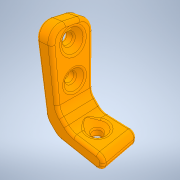
# Autodesk Inventor part: Уголок
Saved by Autodesk Inventor 2021.1 (Build 251245010, 245A)
## iProperties
Created: 2026-06-28
Part Number: Уголок
Material: Типовые
Document SubType Name: Modeling
Designer: Андрей Тарасов
Density: 1 g/cm^3
Appearance: По умолчанию
Author: Андрей Тарасов
Autodesk Inventor part; units mm, degrees
ref_plane "YZ Plane" through (0, 0, 0) normal (1, 0, 0) x (0, 1, 0)
ref_plane "XZ Plane" through (0, 0, 0) normal (0, 1, 0) x (-1, 0, 0)
ref_plane "XY Plane" through (0, 0, 0) normal (0, 0, 1) x (1, 0, 0)
sketch "Эскиз1" plane through (0, 0, 0) normal (0, 0, 1) x (1, 0, 0)
  line L0 (0, 30) -> (0, 0)
  line L1 (0, 0) -> (20, 0)
  line L2 (20, 0) -> (20, 5)
  line L3 (20, 5) -> (5, 5)
  line L4 (5, 5) -> (5, 30)
  line L5 (5, 30) -> (0, 30)
  line L6 (0, 25) -> (5, 25) construction
  line L7 (0, 15) -> (5, 15) construction
  point P0 (0, 0)
  dimension "d0" = 30
  dimension "d1" = 15
  dimension "d2" = 10
  dimension "d3" = 20
  dimension "d4" = 5
  dimension "d5" = 5
  constraints: 16 end point, 5 perpendicular, 3 point on line, 2 horizontal, 1 coincident, 1 midpoint, 1 parallel
  measures "d0" distance between parallel lines of L1 L5
  measures "d1" distance between parallel lines of L1 L7
  measures "d2" distance between parallel lines of L6 L7
  measures "d3" distance between parallel lines of L2 L0
  measures "d4" distance between parallel lines of L3 L1
  measures "d5" distance between parallel lines of L4 L0
extrude "Выдавливание1" add sketch "Эскиз1" along normal blind 12
sketch "Эскиз2" plane through (0, 0, 0) normal (-1, 0, 0) x (0, 0, 1)
  line L0 (0, 30) -> (12, 30) projected
  line L1 (6, 30) -> (6, 0) construction
  line L2 (0, 0) -> (12, 0) projected
  circle A0 centre (6, 15.3) radius 1.6
  circle A1 centre (6, 25.3) radius 1.6
  dimension "d8" = 3.2
  dimension "d9" = 10
  dimension "d10" = 15.3
  constraints: 2 centre point, 2 end point, 2 midpoint, 2 point on line, 1 equal radius
  measures "d8" diameter of A0
  measures "d9" distance of A0.centre A1.centre
  measures "d10" distance from line of L2 A0.centre
extrude "Выдавливание2" cut sketch "Эскиз2" against normal up to surface (5 mm away)
sketch "Эскиз3" plane through (5, 5, 0) normal (0, 1, 0) x (1, 0, 0)
  circle A0 centre (7.5, -6) radius 1.6
  line L0 (0, 0) -> (0, -12) projected
  line L1 (0, -6) -> (15, -6) construction
  line L2 (15, 0) -> (15, -12) projected
  point P0 (-5, 0)
  dimension "d22" = 3.2
  constraints: 3 midpoint, 2 end point, 1 centre point
  measures "d22" diameter of A0
extrude "Выдавливание3" cut sketch "Эскиз3" against normal up to surface (5 mm away)
chamfer "Фаска1" distance 1.8 angle 45 3 edges at (5, 25.3, 4.4) (5, 15.3, 4.4) (10.9, 5, 6)
chamfer "Фаска2" distance 4 angle 45 2 edges at (5, 5, 6) (0, 0, 6)
fillet "Сопряжение1" radius 4 6 edges at (2.5, 30, 12) (2.5, 30, 0) (0, 4, 6) (4, 0, 6) (5, 9, 6) (9, 5, 6)
fillet "Сопряжение1" radius 2 2 edges at (20, 5, 6) (20, 0, 6)
fillet "Сопряжение2" radius 1 37 edges at (3.2, 25.3, 4.4) (0, 25.3, 4.4) (0, 15.8284, 12) (0.3045, 4.1261, 12) (2, 2, 12) (4.1261, 0.3045, 12) (11.8284, 0, 12) (0, 30, 6) (0, 28.8284, 1.1716) (0, 15.8284, 0) (0.3045, 4.1261, 0) (2, 2, 0) (4.1261, 0.3045, 0) (11.8284, 0, 0) (0, 28.8284, 10.8284) (0, 15.3, 4.4) (3.2, 15.3, 4.4) (5, 25.3, 2.6) (5, 15.3, 2.6) (5, 28.8284, 1.1716) (5, 30, 6) (5, 28.8284, 10.8284) (5, 18.3284, 12) (2.5, 26, 12) (7, 7, 12) (19.4142, 4.4142, 12) (14.3284, 5, 12) (2.5, 26, 0) (7, 7, 0) (19.4142, 4.4142, 0) (14.3284, 5, 0) (5, 18.3284, 0) (10.9, 0, 6) (10.9, 3.2, 6) (8.4117, 5.6895, 6.0997) (14.1269, 5, 3.0145) (14.1269, 5, 8.9855)
equation "\"d5\" = d4"
